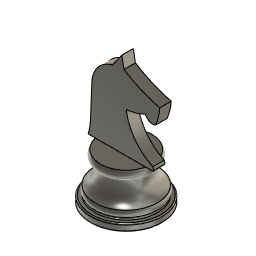
kn (Autodesk Fusion 360 design; units mm, degrees)
Autodesk Fusion 360 part; units mm, degrees
sketch "Sketch1" plane through (0, 0, 0) normal (0, 1, 0) x (1, 0, 0)
  arc A0 (10.9532, 18.2143) -> (7.4805, 11.2112) centre (14.3558, 12.1645) ccw
  arc A1 (10.9532, 18.2143) -> (10.9532, 20.4137) centre (9.6107, 19.314) ccw
  arc A2 (10.9532, 21.1945) -> (10.9532, 20.4137) centre (10.8577, 20.8041) ccw
  line L0 (10.9532, 21.1945) -> (12.1042, 21.1945)
  line L1 (12.5136, 21.6039) -> (12.5136, 23.3712)
  arc A3 (12.1042, 21.1945) -> (12.5136, 21.6039) centre (12.1042, 21.6039) ccw
  arc A4 (12.5136, 23.3712) -> (12.1666, 23.7182) centre (12.1666, 23.3712) ccw
  arc A5 (9, 7.5) -> (7.4805, 11.2112) centre (7.3256, 8.9811) ccw
  line L2 (9, 7.5) -> (0, 7.5)
  line L3 (12.1666, 23.7182) -> (0, 23.7182)
  line L4 (0, 23.7182) -> (0, 7.5)
  line L5 (0.6, 23.3) -> (11.6973, 23.3693)
  line L6 (12.0014, 23.0689) -> (12.0095, 21.7682)
  line L7 (11.7426, 21.5014) -> (11.0004, 21.5063)
  arc A6 (8.9, 8) -> (7.5, 10.9) centre (7.3853, 9.0567) ccw
  line L8 (7.5, 10.9) -> (7.2, 10.9)
  arc A7 (10.5, 18.5) -> (7.2, 10.9) centre (14.3054, 12.3312) ccw
  arc A8 (10.5, 18.5) -> (10.5, 20.2143) centre (9.62, 19.3571) ccw
  arc A9 (11.0004, 21.5063) -> (10.5, 20.2143) centre (10.9054, 20.8002) ccw
  arc A10 (11.7426, 21.5014) -> (12.0095, 21.7682) centre (11.7443, 21.7666) ccw
  arc A11 (12.0014, 23.0689) -> (11.6973, 23.3693) centre (11.6991, 23.067) ccw
  line L9 (8.9, 8) -> (9, 7.5)
  line L10 (0.6, 23.3) -> (0, 23.3)
  constraint horizontal L0
  constraint perpendicular L0 L1
  constraint tangent L0 A3
  constraint tangent L1 A3
  constraint tangent L1 A4
  constraint horizontal L2
  constraint tangent A4 L3
  constraint perpendicular L1 L3
  constraint perpendicular L2 L4
  constraint perpendicular L5 L6
  constraint horizontal L8
  constraint tangent L7 A10
  constraint tangent L6 A10
  constraint tangent L6 A11
  constraint tangent L5 A11
  constraint coincident L4 L10.end
  constraint perpendicular L4 L10
sketch "Sketch2" plane through (0, 0, 0) normal (0, 1, 0) x (-1, 0, 0)
sketch "Sketch3" plane through (0, 0, 0) normal (0, 1, 0) x (1, 0, 0)
  arc A0 (11.3144, 6.1353) -> (11.3144, 7.5) centre (10.2425, 6.8176) ccw
  arc A1 (11.3144, 6.1353) -> (2, -6.5) centre (18.2039, -8.6943) ccw
  arc A2 (8.6108, -8.4073) -> (2, -6.5) centre (-0.6811, -28.2035) ccw
  arc A3 (10, -7) -> (8.6108, -8.4073) centre (13.739, -12.0803) ccw
  arc A4 (12.3, -7) -> (10, -7) centre (11.15, -9.1166) ccw
  arc A5 (13.739, -12.9224) -> (12.3, -7) centre (-6.7336, -14.7609) ccw
  arc A6 (13.739, -12.9224) -> (1.2183, -18.2658) centre (23.4773, -53.0821) ccw
  line L0 (1.2183, -18.2658) -> (0.4532, -22.2017)
  line L1 (0.4532, -22.2017) -> (-2.729, -17.6495)
  arc A7 (-10, -9) -> (-2.729, -17.6495) centre (-0.4679, -8.3679) ccw
  line L2 (-10, -9) -> (-10.5, 3)
  arc A8 (-10.5, 3) -> (-11.3248, 7.5) centre (-26.9211, 2.3158) ccw
  line L3 (-11.3248, 7.5) -> (11.3144, 7.5)
  constraint tangent L2 A8
  constraint horizontal L3
revolve "Revolve3" add sketch "Sketch1" angle 360 about axis through (0, 0, -23.7182) along (0, 0, 1) makes body 1
extrude "Extrude1" add sketch "Sketch3" along normal blind 4 separate body makes body 2
move_body "Move1" bodies 2 to x (1, 0, 0) y (0, 1, 0) z (0, 0, 1) at (0, -2, 0)
named bodies: "Base", "Profile"
